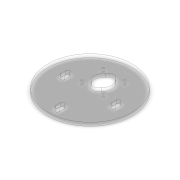
# Autodesk Inventor part: Base Plate
Saved by Autodesk Inventor 2020 (Build 240168000, 168)
## iProperties
Created: 2020-03-27
Part Number: Base Plate
Material: Acrylic
Document SubType Name: Modeling
Designer: chitl
Density: 1.188 g/cm^3
Appearance: Transparent - Clear
Author: chitl
Autodesk Inventor part; units mm, degrees
ref_plane "YZ Plane" through (0, 0, 0) normal (1, 0, 0) x (0, 1, 0)
ref_plane "XZ Plane" through (0, 0, 0) normal (0, 1, 0) x (-1, 0, 0)
ref_plane "XY Plane" through (0, 0, 0) normal (0, 0, 1) x (1, 0, 0)
sketch "Sketch1" plane through (0, 0, 0) normal (0, 1, 0) x (-1, 0, 0)
  line L0 (15.2617, 5.412) -> (-15.7383, 36.412) construction
  line L1 (15.2617, 36.412) -> (-15.7383, 5.412) construction
  line L2 (48.4032, 51.2455) -> (-48.8799, 51.2455) construction
  line L3 (-48.8799, 51.2455) -> (-48.8799, 71.2455) construction
  line L4 (-48.8799, 71.2455) -> (48.4032, 71.2455) construction
  line L5 (48.4032, 71.2455) -> (48.4032, 51.2455) construction
  line L6 (48.4032, 51.2455) -> (-48.8799, 71.2455) construction
  line L7 (-48.8799, 51.2455) -> (48.4032, 71.2455) construction
  line L8 (16.9077, -0.088) -> (-17.3843, -0.088)
  line L9 (-21.2383, 3.766) -> (-21.2383, 38.058)
  line L10 (-17.3843, 41.912) -> (16.9077, 41.912)
  line L11 (20.7617, 38.058) -> (20.7617, 3.766)
  line L12 (20.7617, -0.088) -> (-21.2383, 41.912) construction
  line L13 (-21.2383, -0.088) -> (20.7617, 41.912) construction
  line L14 (20.7617, 3.766) -> (16.9077, -0.088)
  line L15 (-17.3843, -0.088) -> (-21.2383, 3.766)
  line L16 (-17.3843, 41.912) -> (-21.2383, 38.058)
  line L17 (16.9077, 41.912) -> (20.7617, 38.058)
  circle A0 centre (36.4032, 39.2455) radius 12 construction
  circle A1 centre (-36.8799, 39.2455) radius 12 construction
  circle A2 centre (-0.0151, 83.2455) radius 12 construction
  line L18 (-0.2367, 13.9012) -> (-0.24, 27.9229) construction
  line L19 (7.7643, 13.9031) -> (7.761, 27.9248)
  line L20 (-8.241, 27.921) -> (-8.2377, 13.8992)
  arc A3 (-8.2377, 13.8992) -> (7.7643, 13.9031) centre (-0.2367, 13.9012) ccw
  arc A4 (7.761, 27.9248) -> (-8.241, 27.921) centre (-0.24, 27.9229) ccw
  line L21 (36.4032, 35.4355) -> (36.4032, 43.0555) construction
  line L22 (39.1532, 35.4355) -> (39.1532, 43.0555)
  line L23 (33.6532, 43.0555) -> (33.6532, 35.4355)
  arc A5 (33.6532, 35.4355) -> (39.1532, 35.4355) centre (36.4032, 35.4355) ccw
  arc A6 (39.1532, 43.0555) -> (33.6532, 43.0555) centre (36.4032, 43.0555) ccw
  line L24 (-36.8799, 35.4355) -> (-36.8799, 43.0555) construction
  line L25 (-34.1299, 35.4355) -> (-34.1299, 43.0555)
  line L26 (-39.6299, 43.0555) -> (-39.6299, 35.4355)
  arc A7 (-39.6299, 35.4355) -> (-34.1299, 35.4355) centre (-36.8799, 35.4355) ccw
  arc A8 (-34.1299, 43.0555) -> (-39.6299, 43.0555) centre (-36.8799, 43.0555) ccw
  line L27 (-0.0151, 79.4355) -> (-0.0151, 87.0555) construction
  line L28 (2.7349, 79.4355) -> (2.7349, 87.0555)
  line L29 (-2.7651, 87.0555) -> (-2.7651, 79.4355)
  arc A9 (-2.7651, 79.4355) -> (2.7349, 79.4355) centre (-0.0151, 79.4355) ccw
  arc A10 (2.7349, 87.0555) -> (-2.7651, 87.0555) centre (-0.0151, 87.0555) ccw
  ellipse E0 centre (-0.2383, 39.985) end of major axis (-0.2383, 100.7443) minor radius 60.8111
  circle A11 centre (15.2617, 5.412) radius 1.5
  circle A12 centre (-15.7383, 5.412) radius 1.5
  circle A13 centre (-15.7383, 36.412) radius 1.5
  circle A14 centre (15.2617, 36.412) radius 1.5
  circle A15 centre (-0.2383, 20.912) radius 12.5
  point P0 (-0.2383, 61.2455)
  point P1 (-0.2383, 61.2455)
  point P2 (-0.2383, 20.912)
  point P3 (7.1468, 30.9972)
  point P4 (7.1516, 10.8304)
  point P5 (-7.6234, 10.8269)
  point P6 (-7.6283, 30.9936)
  dimension "d45" = 31
  dimension "d46" = 31
  dimension "d47" = 20
  dimension "d48" = 12
  dimension "d49" = 12
  dimension "d50" = 42
  dimension "d51" = 42
  dimension "d52" = 3.854
  dimension "d53" = 45
  dimension "d54" = 3.854
  dimension "d55" = 45
  dimension "d56" = 3.854
  dimension "d57" = 45
  dimension "d58" = 3.854
  dimension "d59" = 45
  dimension "d60" = 12
  dimension "d61" = 16.002
  dimension "d63" = 3.81
  dimension "d64" = 5.5
  dimension "d65" = 3.81
  dimension "d66" = 5.5
  dimension "d67" = 3.81
  dimension "d68" = 5.5
  dimension "d71" = 3
  dimension "d72" = 3
  dimension "d73" = 3
  dimension "d74" = 3
  dimension "d75" = 25
  constraints: 68 end point, 20 tangent, 16 centre point, 16 point on circle, 11 midpoint, 10 coincident, 8 parallel, 8 point on line, 4 vertical alignment, 3 vertical, 2 horizontal, 2 horizontal alignment, 2 perpendicular, 2 other
  measures "d45" distance of L1.end L0.start
  measures "d46" distance of L0.start point (15.262, 36.412)
  measures "d47" distance of L2.end L3.end
  measures "d48" distance from line of point (36.403, 39.246) L2
  measures "d49" distance from line of L2 point (-36.88, 39.246)
  measures "d50" distance of L12.end L13.end
  measures "d51" distance of L13.start L12.end
  measures "d52" distance of L11.end L12.start
  measures "d53" angle of L11 L14
  measures "d54" distance of L8.end L13.start
  measures "d55" angle of L8 L15
  measures "d56" distance of L10.start L12.end
  measures "d57" angle of L10 L16
  measures "d58" distance of L10.end L13.end
  measures "d59" angle of L10 L17
  measures "d60" distance from line of point (-0.015, 83.246) L4
  measures "d61" diameter of A4
  measures "d63" distance of A0.centre L21.end
  measures "d64" diameter of A6
  measures "d65" distance of A1.centre L24.end
  measures "d66" diameter of A8
  measures "d67" distance of A2.centre L27.end
  measures "d68" diameter of A10
  measures "d71" diameter of A11
  measures "d72" diameter of A12
  measures "d73" diameter of A13
  measures "d74" diameter of A14
  measures "d75" diameter of A15
extrude "Extrusion4" add sketch "Sketch1" along normal blind 5 contours L8 L15 L9 L16 L10 L17 L11 L14 | E0
equation "\"d46\" = d45"
equation "\"d49\" = d48"
equation "\"d54\" = d52"
equation "\"d56\" = d54"
equation "\"d57\" = d55"
equation "\"d58\" = d54"
equation "\"d59\" = d55"
equation "\"d60\" = d49"
equation "\"d65\" = d63"
equation "\"d66\" = d64"
equation "\"d67\" = d65"
equation "\"d68\" = d64"
equation "\"d72\" = d71"
equation "\"d73\" = d72"
equation "\"d74\" = d73"
body "Solid2"
